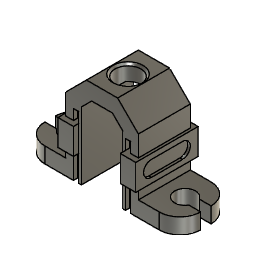
lesson1 v1 (Autodesk Fusion 360 design; units mm, degrees)
Autodesk Fusion 360 part; units mm, degrees
sketch "Sketch1" plane through (0, 0, 0) normal (0, 0, 1) x (1, 0, 0)
  line L0 (75, -25) -> (-75, -25)
  line L1 (-75, -25) -> (-75, 25)
  line L2 (-75, 25) -> (75, 25)
  line L3 (75, 25) -> (75, -25)
  line L4 (75, -25) -> (-75, 25) construction
  line L5 (-75, -25) -> (75, 25) construction
  dimension "d1" = 150
  dimension "d2" = 50
  constraint horizontal L0
  constraint perpendicular L0 L1
  constraint parallel L0 L2
  constraint parallel L1 L3
  constraint coincident L4 origin
  constraint coincident L5 origin
  measures "d1" distance of L1.end L2.end
  measures "d2" distance of L0.end L1.end
extrude "Extrude1" add sketch "Sketch1" along normal blind 15 makes body 1
sketch "Sketch2" plane through (0, 0, 15) normal (0, 0, 1) x (-1, 0, 0)
  line L0 (-75, -25) -> (75, -25)
  line L1 (75, -25) -> (75, 25)
  line L2 (75, 25) -> (-75, 25)
  line L3 (-75, 25) -> (-75, -25)
  line L4 (-25, 25) -> (25, 25)
  line L5 (25, 25) -> (25, -25)
  line L6 (25, -25) -> (-25, -25)
  line L7 (-25, -25) -> (-25, 25)
  line L8 (-25, 25) -> (25, -25) construction
  line L9 (25, 25) -> (-25, -25) construction
  dimension "d5" = 50
  constraint horizontal L4
  constraint perpendicular L4 L5
  constraint parallel L4 L6
  constraint parallel L5 L7
  constraint coincident L8 origin
  constraint coincident L9 origin
  measures "d5" distance of L5.end L6.end
extrude "Extrude2" add sketch "Sketch2" along normal blind 75 contours L0 L2 L4 L5 L6 L7 bodies 1
move_face "OffsetFaces1" offset 10 1 faces at (25, 8.3333, 40) on bodies 1
move_face "OffsetFaces2" offset 10 1 faces at (-25, -8.3333, 40) on bodies 1
fillet "Fillet1" radius 20 4 edges at (-75, 25, 7.5) (-75, -25, 7.5) (75, 25, 7.5) (75, -25, 7.5) on bodies 1
sketch "Sketch3" plane through (0, 0, 15) normal (0, 0, 1) x (-1, 0, 0)
  arc A0 (-55, 25) -> (-75, 5) centre (-55, 5) ccw
  line L0 (-75, 5) -> (-75, -5)
  arc A1 (-75, -5) -> (-55, -25) centre (-55, -5) ccw
  line L1 (-55, -25) -> (-35, -25)
  line L2 (-35, -25) -> (-35, 25)
  line L3 (-35, 25) -> (-55, 25)
  line L4 (-75, 5) -> (-55, 5)
  line L5 (-55, 5) -> (-55, -5)
  line L6 (-55, -5) -> (-75, -5)
  line L7 (0, 0) -> (0, 40) construction
  line L8 (75, 5) -> (55, 5)
  line L9 (55, 5) -> (55, -5)
  line L10 (55, -5) -> (75, -5)
  line L11 (75, 5) -> (75, -5)
  circle A2 centre (-55, 0) radius 10
  circle A3 centre (55, 0) radius 10
  dimension "d12" = 20
  dimension "d13" = 20
  constraint coincident A0.end L0.start
  constraint coincident A0.centre L4.end
  constraint coincident A1.centre L5.end
  constraint coincident L0.end A1.start
  constraint coincident L7.start origin
  constraint perpendicular L3 L7
  constraint symmetric A0.end L7 L8.start
  constraint symmetric A0.centre L7 L8.end
  constraint symmetric A1.centre L7 L9.end
  constraint symmetric L0.end L7 L10.end
  constraint midpoint L5 A2.centre
  constraint midpoint L9 A3.centre
  measures "d12" diameter of A2
  measures "d13" diameter of A3
extrude "Extrude3" cut sketch "Sketch3" against normal blind 30 contours L0 L4 L6 A2 | L4 L5 L6 A2 | L4 L5 L6 A2 | L8 L10 L11 A3 | L8 L9 L10 A3 | L8 L9 L10 A3 bodies 1
sketch "Sketch4" plane through (0, 25, 0) normal (0, 1, 0) x (-1, 0, 0)
  line L0 (-55, 15) -> (-55, 0)
  line L1 (-55, 0) -> (55, 0)
  line L2 (55, 0) -> (55, 15)
  line L3 (55, 15) -> (35, 15)
  line L4 (35, 15) -> (35, 90)
  line L5 (35, 90) -> (-35, 90)
  line L6 (-35, 90) -> (-35, 15)
  line L7 (-35, 15) -> (-55, 15)
  line L8 (20, 15) -> (20, 75)
  line L9 (20, 75) -> (-20, 75)
  line L10 (-20, 75) -> (-20, 15)
  line L11 (-20, 15) -> (-20, 0)
  line L12 (20, 15) -> (20, 0)
  dimension "d16" = -15
  constraint coincident L1 L11.end
  constraint perpendicular L1 L11
  constraint coincident L1 L12.end
  constraint perpendicular L1 L12
extrude "Extrude4" cut sketch "Sketch4" against normal blind 65 contours L1 L8 L9 L10 L11 L12 bodies 1
chamfer "Chamfer1" distance 10 angle 45 2 edges at (20, 0, 75) (-20, 0, 75) on bodies 1
chamfer "Chamfer1" distance 20 angle 45 2 edges at (-35, 0, 90) (35, 0, 90) on bodies 1
sketch "Sketch6" plane through (0, 0, 15) normal (0, 0, 1) x (-1, 0, 0)
  line L0 (-63.6603, -5) -> (-75, -5)
  arc A0 (-75, -5) -> (-55, -25) centre (-55, -5) ccw
  line L1 (-55, -25) -> (-35, -25)
  line L2 (-35, -25) -> (-35, 25)
  line L3 (-35, 25) -> (-55, 25)
  arc A1 (-55, 25) -> (-75, 5) centre (-55, 5) ccw
  line L4 (-75, 5) -> (-63.6603, 5)
  arc A2 (-63.6603, -5) -> (-63.6603, 5) centre (-55, 0) ccw
  line L5 (-35, 25) -> (-30, 25)
  line L6 (-30, 25) -> (-30, 30)
  line L7 (-30, 30) -> (-37.5, 30)
  line L8 (-37.5, 30) -> (-37.5, 0)
  line L9 (-37.5, 0) -> (0, 0) construction
  line L10 (-35, -25) -> (-30, -25)
  line L11 (-30, -25) -> (-30, -30)
  line L12 (-30, -30) -> (-37.5, -30)
  line L13 (-37.5, -30) -> (-37.5, 0)
  dimension "d22" = 7.5
  constraint coincident L2.end L3.start
  constraint perpendicular L2 L5
  constraint perpendicular L3 L6
  constraint perpendicular L6 L7
  constraint perpendicular L7 L8
  constraint coincident L9.end origin
  constraint perpendicular L8 L9
  constraint symmetric L2.end L9 L1.end
  constraint symmetric L5.end L9 L10.end
  constraint symmetric L6.end L9 L11.end
  constraint symmetric L7.end L9 L12.end
  constraint symmetric L8.end L9 L13.end
  measures "d22" distance of L6.end L7.end
extrude "Extrude5" add sketch "Sketch6" along normal blind 25 from surface at 10 separate body contours L1 L2 L3 L8 L13 | L1 L10 L11 L12 L13 | L3 L5 L6 L7 L8 makes body 2
sketch "Sketch7" plane through (37.5, 0, 0) normal (1, 0, 0) x (0, 1, 0)
  line L0 (-30, 25) -> (30, 25)
  line L1 (30, 25) -> (30, 50)
  line L2 (30, 50) -> (-30, 50)
  line L3 (-30, 50) -> (-30, 25)
  line L4 (-15, 30) -> (15, 30)
  arc A0 (15, 30) -> (15, 45) centre (15, 37.5) ccw
  line L5 (15, 45) -> (-15, 45)
  arc A1 (-15, 45) -> (-15, 30) centre (-15, 37.5) ccw
  line L6 (-15, 37.5) -> (15, 37.5) construction
  point P0 (0, 37.5)
  dimension "d26" = 15
  constraint tangent L4 A0
  constraint tangent A0 L5
  constraint parallel L4 L5
  constraint tangent L5 A1
  constraint tangent L4 A1
  constraint perpendicular L1 L6
  constraint midpoint L6 P0
  measures "d26" distance of A0.centre P0
extrude "Extrude6" cut sketch "Sketch7" against normal blind 2.5 contours L4 A0 L5 A1 bodies 2 1
sketch "Sketch10" plane through (0, 25, 0) normal (0, 1, 0) x (-1, 0, 0)
  line L0 (-35, 70) -> (-35, 15)
  line L1 (-35, 15) -> (-55, 15)
  line L2 (-55, 15) -> (-55, 0)
  line L3 (-55, 0) -> (-20, 0)
  line L4 (-20, 0) -> (-20, 65)
  line L5 (-20, 65) -> (-10, 75)
  line L6 (-10, 75) -> (10, 75)
  line L7 (10, 75) -> (20, 65)
  line L8 (20, 65) -> (20, 0)
  line L9 (20, 0) -> (55, 0)
  line L10 (55, 0) -> (55, 15)
  line L11 (55, 15) -> (35, 15)
  line L12 (35, 15) -> (35, 70)
  line L13 (35, 70) -> (15, 90)
  line L14 (15, 90) -> (-15, 90)
  line L15 (-15, 90) -> (-35, 70)
  line L16 (-20, 0) -> (-25, 0)
  line L17 (-25, 0) -> (-25, 60)
  line L18 (-25, 60) -> (-22.5, 60)
  line L19 (-22.5, 60) -> (-22.5, 0)
  line L20 (-25, 60) -> (-27.5, 60)
  line L21 (-27.5, 60) -> (-27.5, 0)
  line L22 (0, 0) -> (0, 60)
  line L23 (-27.5, 0) -> (-25, 0)
  line L24 (22.5, 60) -> (22.5, 0)
  line L25 (25, 60) -> (22.5, 60)
  line L26 (25, 60) -> (27.5, 60)
  line L27 (27.5, 60) -> (27.5, 0)
  line L28 (27.5, 0) -> (25, 0)
  line L29 (20, 0) -> (25, 0)
  dimension "d38" = 2.5
  constraint coincident L3.end L4.start
  constraint coincident L3 L16.end
  constraint perpendicular L4 L16
  constraint perpendicular L3 L17
  constraint perpendicular L17 L18
  constraint midpoint L16 L19.end
  constraint perpendicular L3 L19
  constraint perpendicular L17 L20
  constraint coincident L3 L21.end
  constraint perpendicular L3 L21
  constraint coincident L22.start origin
  constraint vertical L22
  constraint symmetric L3.end L22 L8.end
  constraint symmetric L16.end L22 L28.end
  constraint symmetric L17.end L22 L25.start
  constraint symmetric L18.end L22 L24.start
  constraint symmetric L19.end L22 L24.end
  constraint symmetric L20.end L22 L26.end
  constraint symmetric L21.end L22 L27.end
  measures "d38" distance of L17.end L20.end
extrude "Extrude10" cut sketch "Sketch10" against normal blind 4 contours L3 L17 L20 L21 L23 | L3 L16 L17 L18 L19 | L9 L24 L25 L26 L27 L28 L29 bodies 2 1
sketch "Sketch11" plane through (0, -25, 0) normal (0, -1, 0) x (1, 0, 0)
  line L0 (35, 70) -> (15, 90)
  line L1 (15, 90) -> (-15, 90)
  line L2 (-15, 90) -> (-35, 70)
  line L3 (-35, 70) -> (-35, 15)
  line L4 (-35, 15) -> (-55, 15)
  line L5 (-55, 15) -> (-55, 0)
  line L6 (-55, 0) -> (-20, 0)
  line L7 (-20, 0) -> (-20, 65)
  line L8 (-20, 65) -> (-10, 75)
  line L9 (-10, 75) -> (10, 75)
  line L10 (10, 75) -> (20, 65)
  line L11 (20, 65) -> (20, 0)
  line L12 (20, 0) -> (55, 0)
  line L13 (55, 0) -> (55, 15)
  line L14 (55, 15) -> (35, 15)
  line L15 (35, 15) -> (35, 70)
  line L16 (25, 60) -> (22.5, 60)
  line L17 (25, 60) -> (27.5, 60)
  line L18 (27.5, 60) -> (27.5, 0)
  line L19 (22.5, 60) -> (22.5, 0)
  line L20 (-22.5, 60) -> (-22.5, 0)
  line L21 (-27.5, 60) -> (-27.5, 0)
  line L22 (-25, 60) -> (-27.5, 60)
  line L23 (-25, 60) -> (-22.5, 60)
  line L24 (-27.5, 0) -> (-25, 0)
  line L25 (-20, 0) -> (-25, 0)
  line L26 (20, 0) -> (25, 0)
  line L27 (27.5, 0) -> (25, 0)
  point P0 (-25, 0)
  point P1 (-27.5, 0)
extrude "Extrude11" cut sketch "Sketch11" against normal blind 4 contours L12 L16 L17 L18 L19 L26 L27 | L6 L20 L21 L22 L23 L24 L25 bodies 1 2
move_face "OffsetFaces3" offset 7.5 2 faces at (30, 26.6667, 33.3333) (30, -26.6667, 33.3333) on bodies 2
sketch "Sketch12" plane through (0, 0, 50) normal (0, 0, 1) x (-1, 0, 0)
  line L0 (-35, -25) -> (-35, 25)
  line L1 (-35, 25) -> (-22.5, 25)
  line L2 (-22.5, 25) -> (-22.5, 30)
  line L3 (-22.5, 30) -> (-37.5, 30)
  line L4 (-37.5, 30) -> (-37.5, -30)
  line L5 (-37.5, -30) -> (-22.5, -30)
  line L6 (-22.5, -30) -> (-22.5, -25)
  line L7 (-22.5, -25) -> (-35, -25)
  line L8 (-22.5, 25) -> (-22.5, 21)
  line L9 (-22.5, 21) -> (-27.5, 21)
  line L10 (-27.5, 21) -> (-27.5, 25)
  line L11 (-22.5, -25) -> (-22.5, -21)
  line L12 (-22.5, -21) -> (-27.5, -21)
  line L13 (-27.5, -21) -> (-27.5, -25)
  dimension "d44" = 5
  dimension "d45" = 5
  constraint coincident L1.end L2.start
  constraint perpendicular L1 L8
  constraint perpendicular L2 L9
  constraint coincident L1 L10.end
  constraint perpendicular L1 L10
  constraint coincident L6.end L7.start
  constraint perpendicular L7 L11
  constraint perpendicular L6 L12
  constraint perpendicular L12 L13
  measures "d44" distance of L8.end L9.end
  measures "d45" distance of L11.end L12.end
extrude "Extrude12" add sketch "Sketch12" against normal blind 25 contours L7 L11 L12 L13 | L1 L8 L9 L10 bodies 2
mirror "Mirror1" about plane through (0, 0, 0) normal (1, 0, 0) of bodies 2 makes body 3
sketch "Sketch13" plane through (0, 0, 90) normal (0, 0, 1) x (-1, 0, 0)
  line L0 (-15, 25) -> (-15, -25)
  line L1 (-15, -25) -> (15, -25)
  line L2 (15, -25) -> (15, 25)
  line L3 (15, 25) -> (-15, 25)
  circle A0 centre (0, 0) radius 12.5
  dimension "d50" = 25
  constraint coincident A0.centre origin
  measures "d50" diameter of A0
extrude "Extrude13" cut sketch "Sketch13" against normal blind 25 contours A0 bodies 1
chamfer "Chamfer2" distance 2 angle 45 1 edges at (11.6541, -4.5202, 90) on bodies 1
sketch "Sketch8" plane through (0, 25, 0) normal (0, 1, 0) x (-1, 0, 0)
  line L0 (-35, 50) -> (-30, 50)
  line L1 (-30, 50) -> (-30, 25)
  line L2 (-30, 25) -> (-35, 25)
  line L3 (-35, 25) -> (-35, 15)
  line L4 (-35, 15) -> (-55, 15)
  line L5 (-55, 15) -> (-55, 0)
  line L6 (-55, 0) -> (-20, 0)
  line L7 (-20, 0) -> (-20, 65)
  line L8 (-20, 65) -> (-10, 75)
  line L9 (-10, 75) -> (10, 75)
  line L10 (10, 75) -> (20, 65)
  line L11 (20, 65) -> (20, 0)
  line L12 (20, 0) -> (55, 0)
  line L13 (55, 0) -> (55, 15)
  line L14 (55, 15) -> (35, 15)
  line L15 (35, 15) -> (35, 70)
  line L16 (35, 70) -> (15, 90)
  line L17 (15, 90) -> (-15, 90)
  line L18 (-15, 90) -> (-35, 70)
  line L19 (-35, 70) -> (-35, 50)
  line L20 (-20, 0) -> (-25, 0)
  line L21 (-25, 0) -> (-25, 60)
  line L22 (-25, 60) -> (-27.5, 60)
  line L23 (-27.5, 60) -> (-27.5, 0)
  line L24 (-25, 60) -> (-22.5, 60)
  line L25 (-22.5, 60) -> (-22.5, 0)
  line L26 (-0.1285, 60) -> (0, 0) construction
  line L27 (22.2427, 60.0958) -> (22.4998, 0.0964)
  line L28 (27.2427, 60.1173) -> (27.4997, 0.1178)
  line L29 (24.7427, 60.1066) -> (27.2427, 60.1173)
  line L30 (24.7427, 60.1066) -> (22.2427, 60.0958)
  line L31 (22.4998, 0.0964) -> (27.4997, 0.1178)
  dimension "d29" = 60
  dimension "d30" = 2.5
  dimension "d31" = 2.5
  constraint coincident L6.end L7.start
  constraint coincident L6 L20.end
  constraint perpendicular L7 L20
  constraint perpendicular L20 L21
  constraint perpendicular L21 L22
  constraint perpendicular L22 L23
  constraint perpendicular L21 L24
  constraint midpoint L20 L25.end
  constraint coincident L26.end origin
  constraint symmetric L21.end L26 L29.start
  constraint symmetric L22.end L26 L28.start
  constraint symmetric L23.end L26 L28.end
  constraint symmetric L24.end L26 L27.start
  constraint symmetric L25.end L26 L27.end
  constraint perpendicular L28 L31
  measures "d29" distance of L20.end L21.end
  measures "d30" distance of L21.end L22.end
  measures "d31" distance of L21.end L24.end
extrude "Extrude9" [suppressed]
extrude "Extrude7" [suppressed]
sketch "Sketch9" plane through (0, -25, 0) normal (0, -1, 0) x (1, 0, 0)
  line L0 (35, 25) -> (30, 25)
  line L1 (30, 25) -> (30, 50)
  line L2 (30, 50) -> (35, 50)
  line L3 (35, 50) -> (35, 70)
  line L4 (35, 70) -> (15, 90)
  line L5 (15, 90) -> (-15, 90)
  line L6 (-15, 90) -> (-35, 70)
  line L7 (-35, 70) -> (-35, 15)
  line L8 (-35, 15) -> (-55, 15)
  line L9 (-55, 15) -> (-55, 0)
  line L10 (-55, 0) -> (-20, 0)
  line L11 (-20, 0) -> (-20, 65)
  line L12 (-20, 65) -> (-10, 75)
  line L13 (-10, 75) -> (10, 75)
  line L14 (10, 75) -> (20, 65)
  line L15 (20, 65) -> (20, 0)
  line L16 (20, 0) -> (55, 0)
  line L17 (55, 0) -> (55, 15)
  line L18 (55, 15) -> (35, 15)
  line L19 (35, 15) -> (35, 25)
  line L20 (-22.2427, 60.0958) -> (-22.4998, 0.0964)
  line L21 (-27.2427, 60.1173) -> (-27.4997, 0.1178)
  line L22 (-24.7427, 60.1066) -> (-27.2427, 60.1173)
  line L23 (-24.7427, 60.1066) -> (-22.2427, 60.0958)
  line L24 (25, 60) -> (22.5, 60)
  line L25 (25, 60) -> (27.5, 60)
  line L26 (27.5, 60) -> (27.5, 0)
  line L27 (22.5, 60) -> (22.5, 0)
  line L28 (-27.4997, 0.1178) -> (-22.4998, 0.0964)
  constraint coincident L21.end L28.start
  constraint coincident L20.end L28.end
extrude "Extrude8" [suppressed]
sketch "Sketch5" plane through (0, 0, 90) normal (0, 0, 1) x (-1, 0, 0)
  line L0 (-15, 25) -> (-15, -25)
  line L1 (-15, -25) -> (15, -25)
  line L2 (15, -25) -> (15, 25)
  line L3 (15, 25) -> (-15, 25)
  line L4 (-35, 25) -> (-30, 25)
  line L5 (-30, 25) -> (-30, 30)
  line L6 (-30, 30) -> (-37.5, 30)
  line L7 (-37.5, 30) -> (-37.5, 0)
  line L8 (0, 0) -> (-37.5, 0) construction
  line L9 (-35, -25) -> (-30, -25)
  line L10 (-30, -25) -> (-30, -30)
  line L11 (-30, -30) -> (-37.5, -30)
  line L12 (-37.5, -30) -> (-37.5, 0)
  dimension "d21" = 7.5
  constraint horizontal L4
  constraint perpendicular L4 L5
  constraint perpendicular L5 L6
  constraint perpendicular L6 L7
  constraint coincident L8.start origin
  constraint perpendicular L7 L8
  constraint symmetric L4.start L8 L9.start
  constraint symmetric L4.end L8 L9.end
  constraint symmetric L5.end L8 L10.end
  constraint symmetric L6.end L8 L11.end
  constraint symmetric L7.end L8 L12.end
  measures "d21" distance of L5.end L6.end
